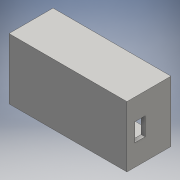
# Autodesk Inventor part: dol
Saved by Autodesk Inventor 2016 SP1 (Build 200210100, 210)
## iProperties
Created: 2019-02-20
Part Number: dol
Material: Ogólny
Document SubType Name: Modeling
Designer: Maciek
Density: 1 g/cm^3
Appearance: Domyślna
Author: Maciek
Autodesk Inventor part; units mm, degrees
ref_plane "YZ Plane" through (0, 0, 0) normal (1, 0, 0) x (0, 1, 0)
ref_plane "XZ Plane" through (0, 0, 0) normal (0, 1, 0) x (-1, 0, 0)
ref_plane "XY Plane" through (0, 0, 0) normal (0, 0, 1) x (1, 0, 0)
sketch "Szkic1" plane through (0, 0, 0) normal (0, 1, 0) x (-1, 0, 0)
  line L0 (0, 0) -> (42.5, 0)
  line L1 (42.5, 0) -> (42.5, 20.5)
  line L2 (42.5, 20.5) -> (0, 20.5)
  line L3 (0, 20.5) -> (0, 0)
  line L4 (42.5, 20.5) -> (44, 20.5) construction
  line L5 (44, 20.5) -> (44, 22) construction
  line L6 (44, 22) -> (-1.5, 22)
  line L7 (-1.5, 22) -> (-1.5, -1.5)
  line L8 (-1.5, -1.5) -> (44, -1.5)
  line L9 (44, -1.5) -> (44, 22)
  line L10 (42.5, 20.5) -> (37.5, 20.5) construction
  line L11 (0, 20.5) -> (5, 20.5) construction
  line L12 (37.5, 20.5) -> (33.5, 20.5)
  line L13 (33.5, 20.5) -> (33.5, 16.5)
  line L14 (33.5, 16.5) -> (37.5, 16.5)
  line L15 (37.5, 16.5) -> (37.5, 20.5)
  line L16 (5, 20.5) -> (9, 20.5)
  line L17 (9, 20.5) -> (9, 16.5)
  line L18 (9, 16.5) -> (5, 16.5)
  line L19 (5, 16.5) -> (5, 20.5)
  line L20 (37.5, 0) -> (33.5, 0)
  line L21 (33.5, 0) -> (33.5, 4)
  line L22 (33.5, 4) -> (37.5, 4)
  line L23 (37.5, 4) -> (37.5, 0)
  line L24 (5, 0) -> (9, 0)
  line L25 (9, 0) -> (9, 4)
  line L26 (9, 4) -> (5, 4)
  line L27 (5, 4) -> (5, 0)
  dimension "d0" = 42.5
  dimension "d1" = 20.5
  dimension "d2" = 1.5
  dimension "d3" = 1.5
  dimension "d4" = 45.5
  dimension "d5" = 23.5
  dimension "d6" = 5
  dimension "d7" = 5
  dimension "d8" = 4
  dimension "d9" = 4
  dimension "d10" = 4
  dimension "d11" = 4
  dimension "d12" = 4
  dimension "d13" = 4
  dimension "d14" = 4
  dimension "d15" = 4
  constraints: 56 end point, 12 parallel, 7 horizontal, 7 perpendicular, 6 point on line
  measures "d0" distance of L2.end L1.end
  measures "d1" distance of L1.end L0.end
  measures "d2" distance of L1.end L4.end
  measures "d3" distance of L4.end L5.end
  measures "d4" distance of L8.end L7.end
  measures "d5" distance of L7.end L6.end
  measures "d6" distance of L1.end L10.end
  measures "d7" distance of L2.end L11.end
  measures "d8" distance of L14.end L13.end
  measures "d9" distance of L13.end L12.end
  measures "d10" distance of L17.end L18.end
  measures "d11" distance of L16.end L17.end
  measures "d12" distance of L21.end L22.end
  measures "d13" distance of L20.end L21.end
  measures "d14" distance of L26.end L25.end
  measures "d15" distance of L25.end L24.end
extrude "Wyciągnięcie proste1" add sketch "Szkic1" along normal blind 1.5 contours L3 L2 L19 L18 L17 L13 L14 L15 L1 L0 L23 L22 L21 L25 L26 L27
sketch "Szkic2" plane through (0, 0, 0) normal (0, -1, 0) x (1, 0, 0)
  line L0 (-5, 4) -> (-5, 0) projected
  line L1 (-5, 0) -> (-9, 0)
  line L2 (-9, 0) -> (-9, 4)
  line L3 (-9, 4) -> (-5, 4)
  line L4 (-5, 4) -> (-5, 0)
  line L5 (-33.5, 0) -> (-33.5, 4) projected
  line L6 (-33.5, 0) -> (-37.5, 0)
  line L7 (-37.5, 0) -> (-37.5, 4)
  line L8 (-37.5, 4) -> (-33.5, 4)
  line L9 (-33.5, 4) -> (-33.5, 0)
  line L10 (-37.5, 20.5) -> (-37.5, 16.5) projected
  line L11 (-33.5, 16.5) -> (-37.5, 16.5)
  line L12 (-37.5, 16.5) -> (-37.5, 20.5)
  line L13 (-37.5, 20.5) -> (-33.5, 20.5)
  line L14 (-33.5, 20.5) -> (-33.5, 16.5)
  line L15 (-5, 16.5) -> (-5, 20.5) projected
  line L16 (-33.5, 20.5) -> (-9, 20.5) projected
  line L17 (-5, 16.5) -> (-9, 16.5)
  line L18 (-9, 16.5) -> (-9, 20.5)
  line L19 (-9, 20.5) -> (-5, 20.5)
  line L20 (-5, 20.5) -> (-5, 16.5)
  point P0 (0, 0)
  constraints: 32 end point, 8 parallel, 4 horizontal, 4 perpendicular
extrude "Wyciągnięcie proste2" add sketch "Szkic2" against normal blind 3
sketch "Szkic3" plane through (0, 0, 0) normal (0, -1, 0) x (1, 0, 0)
  line L0 (-42.5, 0) -> (-42.5, -1.5) construction
  line L1 (-42.5, -1.5) -> (-44, -1.5) construction
  line L2 (-44, -1.5) -> (1.5, -1.5)
  line L3 (1.5, -1.5) -> (1.5, 22)
  line L4 (1.5, 22) -> (-44, 22)
  line L5 (-44, 22) -> (-44, -1.5)
  line L6 (-42.5, 0) -> (0, 0)
  line L7 (0, 0) -> (0, 20.5)
  line L8 (0, 20.5) -> (-42.5, 20.5)
  line L9 (-42.5, 20.5) -> (-42.5, 0)
  dimension "d20" = 1.5
  dimension "d21" = 1.5
  dimension "d22" = 45.5
  dimension "d23" = 23.5
  constraints: 20 end point, 4 parallel, 3 perpendicular, 2 horizontal, 1 vertical
  measures "d20" distance of L0.start L0.end
  measures "d21" distance of L0.end L1.end
  measures "d22" distance of L4.end L3.end
  measures "d23" distance of L3.end L2.end
extrude "Wyciągnięcie proste3" add sketch "Szkic3" against normal blind 17
sketch "Szkic4" plane through (-44, 0, -1.5) normal (-1, 0, 0) x (0, 0, 1)
  line L0 (23.5, 0) -> (0, 0) construction
  line L1 (0, 0) -> (11.75, 0) construction
  line L2 (11.75, 0) -> (11.75, 3) construction
  line L3 (11.75, 3) -> (15.25, 3) construction
  line L4 (15.25, 3) -> (15.25, 7) construction
  line L5 (15.25, 7) -> (8.25, 7)
  line L6 (8.25, 7) -> (8.25, 3)
  line L7 (8.25, 3) -> (15.25, 3)
  line L8 (15.25, 3) -> (15.25, 7)
  point P0 (1.5, 0)
  dimension "d26" = 3
  dimension "d27" = 3.5
  dimension "d28" = 4
  dimension "d29" = 7
  dimension "d30" = 4
  constraints: 16 end point, 3 perpendicular, 2 horizontal, 2 parallel, 1 midpoint
  measures "d26" distance of L1.end L2.end
  measures "d27" distance of L2.end L3.end
  measures "d28" distance of L3.end L4.end
  measures "d29" distance of L7.end L6.end
  measures "d30" distance of L6.end L5.end
extrude "Wyciągnięcie proste4" cut sketch "Szkic4" against normal blind 50
